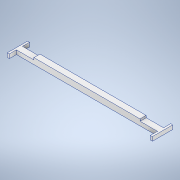
# Autodesk Inventor part: Tbalka760
Saved by Autodesk Inventor 2020.1 (Build 241239000, 239)
## iProperties
Created: 2023-01-06
Part Number: Tbalka760
Material: Алюминий 6061
Document SubType Name: Modeling
Designer: KirikDK
Density: 2.7 g/cm^3
Appearance: Алюминий — плоский
Mass: 1882.44 g
Surface Area: 1022.8 cm^2
Volume: 697.2 cm^3
Author: KirikDK
Autodesk Inventor part; units mm, degrees
ref_plane "YZ Plane" through (0, 0, 0) normal (1, 0, 0) x (0, 1, 0)
ref_plane "XZ Plane" through (0, 0, 0) normal (0, 1, 0) x (-1, 0, 0)
ref_plane "XY Plane" through (0, 0, 0) normal (0, 0, 1) x (1, 0, 0)
sketch "Эскиз1" plane through (0, 0, 0) normal (0, 1, 0) x (-1, 0, 0)
  line L0 (308, 35) -> (-40, 35)
  line L1 (-40, 35) -> (-40, 70)
  line L2 (-40, 70) -> (-50, 70)
  line L3 (-50, 70) -> (-50, -30)
  line L4 (-50, -30) -> (-40, -30)
  line L5 (-40, -30) -> (-40, 5)
  line L6 (-40, 5) -> (308, 5)
  line L7 (308, 5) -> (308, 35)
  line L8 (308, -86) -> (308, -101.2922)
  line L9 (308, 35) -> (656, 35)
  line L10 (656, 35) -> (656, 70)
  line L11 (656, 70) -> (666, 70)
  line L12 (666, 70) -> (666, -30)
  line L13 (666, -30) -> (656, -30)
  line L14 (656, -30) -> (656, 5)
  line L15 (656, 5) -> (308, 5)
  point P0 (0, 0)
  point P1 (616, 0)
  dimension "d0" = 30
  dimension "d1" = 100
  dimension "d2" = 35
  dimension "d3" = 35
  dimension "d4" = 10
  dimension "d5" = 358
  constraints: 32 end point, 7 symmetric about line, 4 perpendicular, 3 point on line, 1 vertical
  measures "d0" distance of L6.end L0.start
  measures "d1" distance of L2.end L3.end
  measures "d2" distance between parallel lines of L4 L6
  measures "d3" distance between parallel lines of L2 L0
  measures "d4" distance of L3.end L4.end
  measures "d5" distance between parallel lines of L7 L3
extrude "Выдавливание1" add sketch "Эскиз1" along normal blind 30
sketch "Эскиз2" plane through (0, 30, 0) normal (0, 1, 0) x (1, 0, 0)
  line L0 (40, -70) -> (50, -70) projected
  line L1 (50, -70) -> (-46, -70)
  line L2 (-46, -70) -> (-46, 30)
  line L3 (-46, 30) -> (50, 30)
  line L4 (50, 30) -> (50, -70)
  line L5 (-666, 30) -> (-666, -70) projected
  line L6 (-666, -70) -> (-570, -70)
  line L7 (-570, -70) -> (-570, 30)
  line L8 (-570, 30) -> (-666, 30)
  line L9 (-666, 30) -> (-666, -70)
  point P0 (0, 0)
  point P1 (40, -70)
  dimension "d8" = 96
  dimension "d9" = 96
  constraints: 16 end point, 4 parallel, 2 horizontal, 2 perpendicular, 1 point on line
  measures "d8" distance between parallel lines of L5 L7
  measures "d9" distance between parallel lines of L2 L4
extrude "Выдавливание2" cut sketch "Эскиз2" against normal blind 10
